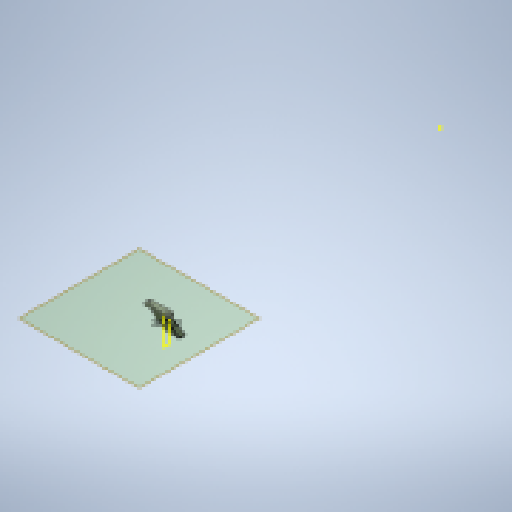
# Autodesk Inventor part: 起落架 新
Saved by Autodesk Inventor 2025.2 (Build 292293000, 293)
## iProperties
Created: 2026-01-24
Part Number: 起落架 新
Material: 常规
Document SubType Name: Modeling
Designer: BO‘S_SLAVE
Density: 1 g/cm^3
Appearance: 默认
Author: BO‘S_SLAVE
Autodesk Inventor part; units mm, degrees
ref_plane "YZ Plane" through (0, 0, 0) normal (1, 0, 0) x (0, 1, 0)
ref_plane "XZ Plane" through (0, 0, 0) normal (0, 1, 0) x (-1, 0, 0)
ref_plane "XY Plane" through (0, 0, 0) normal (0, 0, 1) x (1, 0, 0)
ref_plane "工作平面2" through (-119.683, -39.1814, 539.2089) normal (0, -1, 0) x (-0.0000021, 0, 1)
sketch "草图2" plane through (-119.683, -39.1814, 539.2089) normal (0, -1, 0) x (-0.0000021, 0, 1)
  line L0 (-31, -79.3909) -> (-41, -79.3909)
  line L1 (-41, -79.3909) -> (-41, -36.3909)
  line L2 (-41, -36.3909) -> (-31, -36.3909)
  line L3 (-31, -36.3909) -> (-31, -79.3909)
  circle A0 centre (-36, -74.8909) radius 1.65 projected
  circle A1 centre (-36, -40.8909) radius 1.65 projected
  point P0 (-539.2092, -119.6818)
  point P1 (0, 0)
  dimension "d0" = 10
  dimension "d1" = 43
  dimension "d2" = 5
  dimension "d3" = 4.5
  constraints: 8 end point, 2 parallel, 1 horizontal, 1 perpendicular, 1 other
  measures "d0" distance between parallel lines of L1 L3
  measures "d1" distance between parallel lines of L2 L0
  measures "d2" distance from line of L1 A0.centre
  measures "d3" distance from line of A0.centre L0
extrude "拉伸1" add sketch "草图2" along normal blind 5
ref_plane "工作平面3" through (-119.683, -44.1814, 539.2089) normal (0, -1, 0) x (1, 0, 0.0000021)
sketch "草图4" plane through (-119.683, -44.1814, 539.2089) normal (0, -1, 0) x (1, 0, 0.0000021)
  line L0 (36.3909, -41) -> (79.3909, -41) projected
  line L1 (79.3909, -31) -> (36.3909, -31) projected
  line L2 (71.3909, -41) -> (46.3909, -41)
  line L3 (46.3909, -41) -> (46.3909, -31)
  line L4 (46.3909, -31) -> (71.3909, -31)
  line L5 (71.3909, -31) -> (71.3909, -41)
  line L6 (36.3909, -31) -> (36.3909, -41) projected
  point P0 (119.6818, -539.2092)
  point P1 (71.3909, -31)
  point P2 (46.3909, -41)
  dimension "d10" = 25
  dimension "d11" = 10
  constraints: 8 end point, 2 parallel, 2 point on line, 1 horizontal, 1 perpendicular
  measures "d10" distance between parallel lines of L5 L3
  measures "d11" distance between parallel lines of L6 L3
extrude "拉伸4" add sketch "草图4" along normal blind 50 contours L3 L1 L5 L0
sketch "草图5" plane through (-48.292, -94.1814, 508.2091) normal (1, 0, 0.0000021) x (0.0000021, 0, -1)
  line L0 (0, 50) -> (10, 50) projected
  line L1 (0, 50) -> (0, 0) projected
  line L2 (10, 0) -> (0, 0) projected
  line L3 (10, 50) -> (10, 0) projected
  line L4 (0, 50) -> (28.8675, 0)
  line L5 (28.8675, 0) -> (38.8675, 0)
  line L6 (38.8675, 0) -> (10, 50)
  point P0 (508.2092, 94.1814)
  point P1 (10, 32.6795)
  dimension "d29" = 30
  constraints: 6 end point, 1 collinear, 1 horizontal, 1 parallel
  measures "d29" angle of L1 L4
extrude "拉伸5" add sketch "草图5" against normal blind 25 contours L6 L5 L4 L3
extrude "拉伸6" cut sketch "草图5" against normal blind 25 contours L4 L3 L2 L1
ref_plane "工作平面4" through (-40.292, -44.1814, 508.2091) normal (-0.0000021, 0, 1) x (1, 0, 0.0000021)
sketch "草图7" plane through (-40.292, -44.1814, 508.2091) normal (-0.0000021, 0, 1) x (1, 0, 0.0000021)
  line L0 (-8, 0) -> (-8, -50) projected
  line L1 (-33, 0) -> (-8, 0) projected
  line L2 (-33, -50) -> (-33, 0) projected
  line L3 (-8, -50) -> (-33, -50) projected
  line L4 (-40.6091, 5) -> (-2.3909, 5) projected
  line L5 (-33, 0) -> (-8, 0) projected
  line L6 (0, 0) -> (-8, 0) projected
  line L7 (0, 5) -> (0, 0) projected
  line L8 (0, 5) -> (-43, 5) projected
  line L9 (-43, 5) -> (-43, 0) projected
  line L10 (-33, 0) -> (-43, 0) projected
  line L11 (-8, 0) -> (-33, 0) projected
  line L12 (-33, 0) -> (-8, -50)
  line L13 (-33, -50) -> (-8, 0)
  line L14 (-31.3229, 0) -> (-8, -46.6459)
  line L15 (-33, -3.3541) -> (-9.6771, -50)
  line L16 (-33, -50) -> (-33, 0) projected
  line L17 (-33, -46.6459) -> (-9.6771, 0)
  line L18 (-8, -50) -> (-8, 0) projected
  line L19 (-8, -3.3541) -> (-31.3229, -50)
  line L20 (-30, 0) -> (-30, -50)
  line L21 (-11, -50) -> (-11, 0)
  line L22 (-30, -47.3541) -> (-11, -47.3541)
  line L23 (-30, -2.6459) -> (-11, -2.6459)
  point P0 (40.291, 44.1814)
  point P1 (-33, -46.6459)
  point P2 (-22.1771, -25)
  point P3 (-20.5, -28.3541)
  point P4 (-8, -3.3541)
  point P5 (-18.8229, -25)
  point P6 (-20.5, -21.6459)
  point P7 (-9.6771, 0)
  point P8 (-31.3229, 0)
  point P9 (-11, -40.6459)
  point P10 (-11, -9.3541)
  point P11 (-30, -9.3541)
  point P12 (-30, -40.6459)
  point P13 (-11, -2.6459)
  point P14 (-11, 0)
  point P15 (-30, 0)
  point P16 (-30, -2.6459)
  point P17 (-11, -47.3541)
  point P18 (-30, -47.3541)
  dimension "d44" = 1.5
  dimension "d45" = 1.5
  dimension "d47" = 3
  dimension "d48" = 3
  constraints: 20 end point, 20 point on line, 6 parallel
  measures "d44" distance between parallel lines of L12 L14
  measures "d45" distance between parallel lines of L13 L17
  measures "d47" distance between parallel lines of L2 L20
  measures "d48" distance between parallel lines of L0 L21
extrude "拉伸8" cut sketch "草图7" against normal blind 50 contours L21 L14 L19 | L17 L14 L23 | L22 L19 L15 | L17 L20 L15
ref_plane "工作平面5" through (-48.2919, -94.1814, 469.3416) normal (0, -1, 0) x (1, 0, 0.0000021)
sketch "草图8" plane through (-48.2919, -94.1814, 469.3416) normal (0, -1, 0) x (1, 0, 0.0000021)
  line L0 (0, 10) -> (0, 0) construction
  line L1 (-25, 0) -> (-25, 10) construction
  line L2 (-90, -2.5) -> (65, -2.5)
  line L3 (65, -2.5) -> (65, 12.5)
  line L4 (65, 12.5) -> (-90, 12.5)
  line L5 (-90, 12.5) -> (-90, -2.5)
  line L6 (0, 10) -> (-25, 10) projected
  line L7 (0, 0) -> (-25, 0) projected
  line L8 (0, 10) -> (-25, 10) projected
  line L9 (0, 0) -> (-25, 0) projected
  point P0 (48.291, -469.3417)
  dimension "d40" = 155
  dimension "d41" = 65
  dimension "d49" = 15
  dimension "d50" = 2.5
  constraints: 8 end point, 2 parallel, 1 horizontal, 1 perpendicular
  measures "d40" distance between parallel lines of L3 L5
  measures "d41" distance between parallel lines of L1 L5
  measures "d49" distance between parallel lines of L4 L2
  measures "d50" distance between parallel lines of L7 L2
extrude "拉伸9" add sketch "草图8" along normal blind 5
